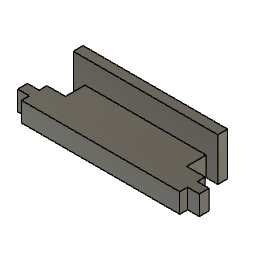
canon_A23_replacement (Autodesk Fusion 360 design; units mm, degrees)
Autodesk Fusion 360 part; units mm, degrees
sketch "Sketch1" plane through (0, 0, 0) normal (0, 0, 1) x (1, 0, 0)
  line L0 (0, 0) -> (46.5, 0)
  line L1 (46.5, 0) -> (46.5, 15)
  line L2 (46.5, 15) -> (0, 15)
  line L3 (0, 15) -> (0, 0)
  dimension "d1" = 46.5
  dimension "d2" = 15
  constraint horizontal L0
  constraint vertical L1
  constraint horizontal L2
  constraint vertical L3
  constraint coincident L0.start L3.end
  measures "d1" distance of L0.start L0.end
  measures "d2" distance of L0.end L1.end
extrude "Extrude1" add sketch "Sketch1" along normal blind 11.5
sketch "Sketch2" plane through (0, 0, 11.5) normal (0, 0, 1) x (-1, 0, 0)
  line L0 (0, -15) -> (0, 0)
  line L1 (0, 0) -> (-46.5, 0)
  line L2 (-46.5, 0) -> (-46.5, -15)
  line L3 (-46.5, -15) -> (0, -15)
  line L4 (0, -15) -> (-4.75, -15)
  line L5 (-4.75, -15) -> (-4.75, -12.5)
  line L6 (-4.75, -12.5) -> (0, -12.5)
  line L7 (0, -12.5) -> (0, -15)
  dimension "d5" = 4.75
  dimension "d6" = 2.5
  constraint horizontal L4
  constraint vertical L5
  constraint horizontal L6
  constraint vertical L7
  constraint coincident L0.start L3.end
  measures "d5" distance of L0.start L4.end
  measures "d6" distance of L4.end L5.end
extrude "Extrude2" cut sketch "Sketch2" against normal blind 11.5 contours L0 L3 L4 L5 L6 L7
sketch "Sketch4" plane through (0, 0, 11.5) normal (0, 0, 1) x (-1, 0, 0)
  line L0 (-4.75, -12.5) -> (0, -12.5)
  line L1 (0, -12.5) -> (0, 0)
  line L2 (0, 0) -> (-46.5, 0)
  line L3 (-46.5, 0) -> (-46.5, -15)
  line L4 (-46.5, -15) -> (-4.75, -15)
  line L5 (-4.75, -15) -> (-4.75, -12.5)
  line L6 (-46.5, -15) -> (-41.75, -15)
  line L7 (-41.75, -15) -> (-41.75, -12.5)
  line L8 (-41.75, -12.5) -> (-46.5, -12.5)
  line L9 (-46.5, -12.5) -> (-46.5, -15)
  dimension "d11" = 4.75
  dimension "d12" = 2.5
  constraint horizontal L6
  constraint vertical L7
  constraint horizontal L8
  constraint vertical L9
  constraint coincident L3.end L4.start
  measures "d11" distance of L3.end L6.end
  measures "d12" distance of L3.end L8.end
extrude "Extrude3" cut sketch "Sketch4" against normal blind 11.5 contours L3 L4 L6 L7 L8 L9
sketch "Sketch5" plane through (0, 0, 11.5) normal (0, 0, 1) x (-1, 0, 0)
  line L0 (-41.75, -12.5) -> (-41.75, -15)
  line L1 (-41.75, -15) -> (-4.75, -15)
  line L2 (-4.75, -15) -> (-4.75, -12.5)
  line L3 (-4.75, -12.5) -> (0, -12.5)
  line L4 (0, -12.5) -> (0, 0)
  line L5 (0, 0) -> (-46.5, 0)
  line L6 (-46.5, 0) -> (-46.5, -12.5)
  line L7 (-46.5, -12.5) -> (-41.75, -12.5)
  line L8 (0, -12.5) -> (-4.75, -12.5)
  line L9 (-4.75, -12.5) -> (-4.75, -2.5)
  line L10 (-4.75, -2.5) -> (0, -2.5)
  line L11 (0, -2.5) -> (0, -12.5)
  dimension "d15" = 10
  constraint horizontal L8
  constraint vertical L9
  constraint horizontal L10
  constraint vertical L11
  constraint coincident L3.end L4.start
  measures "d15" distance of L2.end L9.end
extrude "Extrude4" cut sketch "Sketch5" against normal blind 11.5 contours L3 L4 L8 L9 L10 L11
sketch "Sketch7" plane through (0, 0, 11.5) normal (0, 0, 1) x (-1, 0, 0)
  line L0 (-4.75, -2.5) -> (0, -2.5)
  line L1 (0, -2.5) -> (0, 0)
  line L2 (0, 0) -> (-46.5, 0)
  line L3 (-46.5, 0) -> (-46.5, -12.5)
  line L4 (-46.5, -12.5) -> (-41.75, -12.5)
  line L5 (-41.75, -12.5) -> (-41.75, -15)
  line L6 (-41.75, -15) -> (-4.75, -15)
  line L7 (-4.75, -15) -> (-4.75, -2.5)
  line L8 (-41.75, -12.5) -> (-46.5, -12.5)
  line L9 (-46.5, -12.5) -> (-46.5, -2.5)
  line L10 (-46.5, -2.5) -> (-41.75, -2.5)
  line L11 (-41.75, -2.5) -> (-41.75, -12.5)
  dimension "d18" = 10
  constraint horizontal L8
  constraint vertical L9
  constraint horizontal L10
  constraint vertical L11
  constraint coincident L4.end L5.start
  measures "d18" distance of L4.end L10.end
extrude "Extrude5" cut sketch "Sketch7" against normal blind 11.5 contours L3 L4 L8 L9 L10 L11
sketch "Sketch8" plane through (0, 0, 11.5) normal (0, 0, 1) x (-1, 0, 0)
  line L0 (-41.75, -2.5) -> (-41.75, -15)
  line L1 (-41.75, -15) -> (-4.75, -15)
  line L2 (-4.75, -15) -> (-4.75, -2.5)
  line L3 (-4.75, -2.5) -> (0, -2.5)
  line L4 (0, -2.5) -> (0, 0)
  line L5 (0, 0) -> (-46.5, 0)
  line L6 (-46.5, 0) -> (-46.5, -2.5)
  line L7 (-46.5, -2.5) -> (-41.75, -2.5)
  line L8 (-4.75, -2.5) -> (-7.75, -2.5)
  line L9 (-7.75, -2.5) -> (-7.75, -12.5)
  line L10 (-7.75, -12.5) -> (-4.75, -12.5)
  line L11 (-4.75, -12.5) -> (-4.75, -2.5)
  dimension "d21" = 3
  dimension "d22" = 10
  constraint horizontal L8
  constraint vertical L9
  constraint horizontal L10
  constraint vertical L11
  constraint coincident L2.end L3.start
  measures "d21" distance of L2.end L8.end
  measures "d22" distance of L2.end L10.end
extrude "Extrude6" cut sketch "Sketch8" against normal blind 11.5 contours L2 L8 L9 L10 L11
sketch "Sketch9" plane through (0, 0, 11.5) normal (0, 0, 1) x (-1, 0, 0)
  line L0 (-4.75, -12.5) -> (-7.75, -12.5)
  line L1 (-7.75, -12.5) -> (-7.75, -2.5)
  line L2 (-7.75, -2.5) -> (0, -2.5)
  line L3 (0, -2.5) -> (0, 0)
  line L4 (0, 0) -> (-46.5, 0)
  line L5 (-46.5, 0) -> (-46.5, -2.5)
  line L6 (-46.5, -2.5) -> (-41.75, -2.5)
  line L7 (-41.75, -2.5) -> (-41.75, -15)
  line L8 (-41.75, -15) -> (-4.75, -15)
  line L9 (-4.75, -15) -> (-4.75, -12.5)
  line L10 (-41.75, -2.5) -> (-38.75, -2.5)
  line L11 (-38.75, -2.5) -> (-38.75, -12.5)
  line L12 (-38.75, -12.5) -> (-41.75, -12.5)
  line L13 (-41.75, -12.5) -> (-41.75, -2.5)
  dimension "d25" = 3
  dimension "d26" = 10
  constraint horizontal L10
  constraint vertical L11
  constraint horizontal L12
  constraint vertical L13
  constraint coincident L6.end L7.start
  measures "d25" distance of L6.end L10.end
  measures "d26" distance of L6.end L12.end
extrude "Extrude7" cut sketch "Sketch9" against normal blind 11.5 contours L7 L10 L11 L12 L13
sketch "Sketch10" plane through (0, 0, 11.5) normal (0, 0, 1) x (-1, 0, 0)
  line L0 (-46.5, -2.5) -> (-38.75, -2.5)
  line L1 (-38.75, -2.5) -> (-38.75, -12.5)
  line L2 (-38.75, -12.5) -> (-41.75, -12.5)
  line L3 (-41.75, -12.5) -> (-41.75, -15)
  line L4 (-41.75, -15) -> (-4.75, -15)
  line L5 (-4.75, -15) -> (-4.75, -12.5)
  line L6 (-4.75, -12.5) -> (-7.75, -12.5)
  line L7 (-7.75, -12.5) -> (-7.75, -2.5)
  line L8 (-7.75, -2.5) -> (0, -2.5)
  line L9 (0, -2.5) -> (0, 0)
  line L10 (0, 0) -> (-46.5, 0)
  line L11 (-46.5, 0) -> (-46.5, -2.5)
  line L12 (0, 0) -> (-46.5, 0)
  line L13 (-46.5, 0) -> (-46.5, -12.5)
  line L14 (-46.5, -12.5) -> (0, -12.5)
  line L15 (0, -12.5) -> (0, 0)
  dimension "d29" = 46.5
  constraint horizontal L12
  constraint vertical L13
  constraint horizontal L14
  constraint vertical L15
  constraint coincident L9.end L10.start
  measures "d29" distance of L9.end L10.end
extrude "Extrude8" cut sketch "Sketch10" against normal blind 3.5 contours L0 L1 L7 L8 L9 L10 L11 L12 L13 L14 L15
sketch "Sketch11" plane through (0, 0, 0) normal (0, 0, -1) x (1, 0, 0)
  line L0 (38.75, -2.5) -> (46.5, -2.5)
  line L1 (46.5, -2.5) -> (46.5, 0)
  line L2 (46.5, 0) -> (0, 0)
  line L3 (0, 0) -> (0, -2.5)
  line L4 (0, -2.5) -> (7.75, -2.5)
  line L5 (7.75, -2.5) -> (7.75, -12.5)
  line L6 (7.75, -12.5) -> (4.75, -12.5)
  line L7 (4.75, -12.5) -> (4.75, -15)
  line L8 (4.75, -15) -> (41.75, -15)
  line L9 (41.75, -15) -> (41.75, -12.5)
  line L10 (41.75, -12.5) -> (38.75, -12.5)
  line L11 (38.75, -12.5) -> (38.75, -2.5)
  line L12 (0, 0) -> (46.5, 0)
  line L13 (46.5, 0) -> (46.5, -12.5)
  line L14 (46.5, -12.5) -> (0, -12.5)
  line L15 (0, -12.5) -> (0, 0)
  dimension "d32" = 46.5
  dimension "d33" = 12.5
  constraint horizontal L12
  constraint vertical L13
  constraint horizontal L14
  constraint vertical L15
  constraint coincident L2.end L3.start
  measures "d32" distance of L2.end L1.end
  measures "d33" distance of L2.end L14.end
extrude "Extrude9" cut sketch "Sketch11" against normal blind 3.5 contours L0 L1 L2 L3 L4 L5 L11 L12 L13 L14 L15
extrude "Extrude10" add 1 faces at (18.0833, 9.1667, 3.5) along direction (0, 0, -1) blind 3.5
extrude "Extrude11" cut 1 faces at (28.4167, 5.8333, 8) along direction (0, 0, -1) blind 3.5
extrude "Extrude12" add 1 faces at (18.0833, 12.5, 9.1667) along direction (0, -1, 0) blind 3
extrude "Extrude13" cut 1 faces at (29.4167, 15, 3.8333) along direction (0, -1, 0) blind 3
extrude "Extrude14" add 1 faces at (29.4167, 10.3333, 11.5) along direction (0, 0, 1) blind 1
extrude "Extrude15" add 1 faces at (17.0833, 12, 8.3333) along direction (0, 1, 0) blind 0.5
extrude "Extrude16" cut 1 faces at (17.0833, 11.5, 12.5) along direction (0, 0, -1) blind 0.5
extrude "Extrude17" add 1 faces at (31, 0, 3) along direction (0, -1, 0) blind 1
extrude "Extrude18" cut 1 faces at (31, -1, 3) along direction (0, 1, 0) blind 0.5
extrude "Extrude19" add 1 faces at (18.0833, 7.1667, 4.5) along direction (0, 0, 1) blind 0.5
sketch "Sketch12" plane through (38.75, 0, 0) normal (1, 0, 0) x (0, 1, 0)
  line L0 (9.5, 0) -> (9.5, 5)
  line L1 (9.5, 5) -> (2.5, 5)
  line L2 (2.5, 5) -> (2.5, 0)
  line L3 (2.5, 0) -> (9.5, 0)
  line L4 (2.5, 5) -> (4.5, 5)
  line L5 (4.5, 5) -> (4.5, 0)
  line L6 (4.5, 0) -> (2.5, 0)
  line L7 (2.5, 0) -> (2.5, 5)
  dimension "d56" = 2
  constraint horizontal L4
  constraint vertical L5
  constraint horizontal L6
  constraint vertical L7
  constraint coincident L1.end L2.start
  measures "d56" distance of L1.end L4.end
extrude "Extrude20" add sketch "Sketch12" along normal blind 4.75 contours L1 L2 L3 L4 L5 L6 L7
sketch "Sketch13" plane through (7.75, 0, 0) normal (-1, 0, 0) x (0, -1, 0)
  line L0 (-9.5, 5) -> (-9.5, 0)
  line L1 (-9.5, 0) -> (-2.5, 0)
  line L2 (-2.5, 0) -> (-2.5, 5)
  line L3 (-2.5, 5) -> (-9.5, 5)
  line L4 (-2.5, 5) -> (-4.5, 5)
  line L5 (-4.5, 5) -> (-4.5, 0)
  line L6 (-4.5, 0) -> (-2.5, 0)
  line L7 (-2.5, 0) -> (-2.5, 5)
  dimension "d59" = 2
  constraint horizontal L4
  constraint vertical L5
  constraint horizontal L6
  constraint vertical L7
  constraint coincident L2.end L3.start
  measures "d59" distance of L2.end L4.end
extrude "Extrude21" add sketch "Sketch13" along normal blind 4.75 contours L1 L2 L3 L4 L5 L6 L7
sketch "Sketch14" plane through (0, -0.5, 0) normal (0, -1, 0) x (1, 0, 0)
  line L0 (0, 5) -> (0, 0)
  line L1 (0, 0) -> (46.5, 0)
  line L2 (46.5, 0) -> (46.5, 5)
  line L3 (46.5, 5) -> (0, 5)
  line L4 (3, 0) -> (43.5, 0)
  line L5 (43.5, 0) -> (43.5, 5)
  line L6 (43.5, 5) -> (3, 5)
  line L7 (3, 5) -> (3, 0)
  dimension "d62" = 40.5
  dimension "d63" = 3
  constraint horizontal L4
  constraint vertical L5
  constraint horizontal L6
  constraint vertical L7
  constraint coincident L1 L4.start
  measures "d62" distance of L4.start L4.end
  measures "d63" distance of L0 L7
extrude "Extrude22" add sketch "Sketch14" along normal blind 2 contours L1 L3 L4 L5 L6 L7
extrude "Extrude23" cut 1 faces at (17.0833, 11.5, 12) along direction (0, 0, -1) blind 1
extrude "Extrude24" cut 1 faces at (29.4167, 12.5, 7.3333) along direction (0, -1, 0) blind 0.5
extrude "Extrude25" cut 1 faces at (45.5, -0.5, 3.3333) along direction (0, 1, 0) blind 0.5
extrude "Extrude26" cut 1 faces at (16.5, -2.5, 3.3333) along direction (0, 1, 0) blind 0.5
extrude "Extrude27" cut 1 faces at (1, -0.5, 3.3333) along direction (0, 1, 0) blind 0.5
